Baseboard end stop (Autodesk Fusion 360 design; units mm, degrees)
Autodesk Fusion 360 part; units mm, degrees
sketch "Sketch1" plane through (0, 0, 0) normal (0, 0, 1) x (1, 0, 0)
  line L0 (0, 0) -> (85, 0)
  line L1 (85, 0) -> (85, 10)
  line L2 (85, 10) -> (0, 10)
  line L3 (0, 10) -> (0, 0)
  dimension "d1" = 85
  dimension "d2" = 10
  constraint horizontal L0
  constraint vertical L1
  constraint horizontal L2
  constraint vertical L3
  constraint coincident L0.start L3.end
  measures "d1" distance of L0.start L0.end
  measures "d2" distance of L0.start L2.end
sketch "Sketch2" plane through (0, 0, 0) normal (0, 0, 1) x (1, 0, 0)
  line L0 (-0.1614, 75.5661) -> (84.7889, 75.5661)
  line L1 (84.7889, 75.5661) -> (84.7889, 51.9288)
  line L2 (84.7889, 51.9288) -> (-0.1614, 51.9288)
  line L3 (-0.1614, 51.9288) -> (-0.1614, 75.5661)
  line L4 (101.1356, 28.4435) -> (146.0932, 28.5966)
  spline S0 degree 2 poles (146.0932, 28.5966) (146.4207, 28.6282) (146.6949, 28.9321) knots 0 0 0 1 1 1
  spline S1 degree 2 poles (146.6949, 28.9321) (146.9692, 29.236) (147.6482, 30.13) knots 0 0 0 1 1 1
  spline S2 degree 2 poles (147.6482, 30.13) (148.1849, 30.9015) (149.5583, 30.5785) knots 0 0 0 1 1 1
  spline S3 degree 2 poles (149.5583, 30.5785) (153.6429, 28.642) (156.9825, 32.6978) knots 0 0 0 1 1 1
  line L5 (156.9825, 32.6978) -> (157.6246, 33.353)
  spline S4 degree 2 poles (157.6246, 33.353) (160.1812, 36.1272) (164.5464, 34.2758) knots 0 0 0 1 1 1
  spline S5 degree 2 poles (164.5464, 34.2758) (165.5295, 33.8381) (166.3419, 34.2776) knots 0 0 0 1 1 1
  spline S6 degree 2 poles (166.3419, 34.2776) (166.8177, 34.5478) (167.1305, 34.8437) knots 0 0 0 1 1 1
  spline S7 degree 2 poles (167.1305, 34.8437) (167.4433, 35.1397) (168.5542, 36.1845) knots 0 0 0 1 1 1
  line L6 (168.5542, 36.1845) -> (169.6479, 37.2491)
  spline S8 degree 2 poles (169.6479, 37.2491) (170.01, 37.4964) (170.1507, 38.2343) knots 0 0 0 1 1 1
  spline S9 degree 2 poles (170.1507, 38.2343) (170.2914, 38.9722) (171.1167, 45.0927) knots 0 0 0 1 1 1
  spline S10 degree 2 poles (171.1167, 45.0927) (171.1842, 46.5468) (169.5755, 46.506) knots 0 0 0 1 1 1
  spline S11 degree 2 poles (169.5755, 46.506) (167.9668, 46.4652) (164.4434, 46.4273) knots 0 0 0 1 1 1
  line L7 (164.4434, 46.4273) -> (128.4167, 45.746)
  line L8 (128.4167, 45.746) -> (101.2514, 45.4119)
  line L9 (101.2514, 45.4119) -> (101.1356, 28.4435)
extrude "Extrude1" add sketch "Sketch2" along normal blind 1 contours L4 S0 S1 S2 S3 L5 S4 S5 S6 S7 L6 S8 S9 S10 S11 L7 L8 L9
